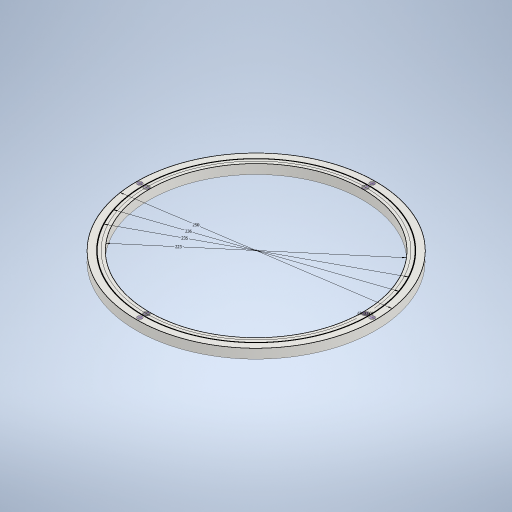
# Autodesk Inventor part: bearing_table
Saved by Autodesk Inventor 2023 (Build 270158000, 158)
## iProperties
Created: 2023-03-04
Part Number: bearing_table
Material: Generic
Document SubType Name: Modeling
Designer: caleb
Density: 1 g/cm^3
Appearance: Default
Author: caleb
Autodesk Inventor part; units mm, degrees
ref_plane "YZ Plane" through (0, 0, 0) normal (1, 0, 0) x (0, 1, 0)
ref_plane "XZ Plane" through (0, 0, 0) normal (0, 1, 0) x (-1, 0, 0)
ref_plane "XY Plane" through (0, 0, 0) normal (0, 0, 1) x (1, 0, 0)
sketch "Sketch1" plane through (0, 0, 0) normal (0, 1, 0) x (-1, 0, 0)
  circle A0 centre (0, 0) radius 111.5
  circle A1 centre (0, 0) radius 125
  circle A2 centre (0, 0) radius 117.5
  circle A3 centre (0, 0) radius 118
  point P0 (-121.5, 0)
  point P1 (-114.5, 0)
  point P2 (0, -114.5)
  point P3 (0, -121.5)
  point P4 (114.5, 0)
  point P5 (121.5, 0)
  point P6 (0, 114.5)
  point P7 (0, 121.5)
  dimension "d0" = 223
  dimension "d1" = 250
  dimension "d2" = 235
  dimension "d3" = 236
  dimension "d16" = 360
  constraints: 4 centre point, 4 coincident, 9 other
  measures "d0" diameter of A0
  measures "d1" diameter of A1
  measures "d2" diameter of A2
  measures "d3" diameter of A3
extrude "Extrusion1" add sketch "Sketch1" against normal blind 10
hole "Hole1" at (114.5, 0, 0) at (0, 0, -114.5) at (-114.5, 0, 0) at (0, 0, 114.5) direction (0, -1, 0) diameter 5 end through all countersink diameter 5.9 countersink angle 90
sketch "Sketch2" plane through (0, -10, 0) normal (0, -1, 0) x (1, 0, 0)
  point P0 (0, 0)
  point P1 (121.5, 0)
  point P2 (0, 121.5)
  point P3 (-121.5, 0)
  point P4 (0, -121.5)
hole "Hole2" at (0, -10, -121.5) at (-121.5, -10, 0) at (0, -10, 121.5) at (121.5, -10, 0) direction (0, 1, 0) diameter 5 end through all countersink diameter 5.9 countersink angle 90
body "Solid1"
